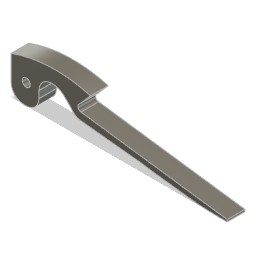
Fork v1 v14 (Autodesk Fusion 360 design; units mm, degrees)
Autodesk Fusion 360 part; units mm, degrees
derive "DerivedContext1" from "Forkzin v1"
sketch "Esboço1" plane through (0, 0, 0) normal (0, 1, 0) x (1, 0, 0)
  line L0 (0, 0) -> (100, 0)
  line L1 (100, 0) -> (100, 10)
  line L2 (100, 10) -> (0, 10)
  line L3 (0, 10) -> (0, 0)
  dimension "d1" = 100
  dimension "d2" = 10
  constraint horizontal L0
  constraint vertical L1
  constraint horizontal L2
  constraint vertical L3
  constraint coincident L0.start L3.end
  measures "d1" distance of L0.start L0.end
  measures "d2" distance of L0.start L2.end
extrude "Extrusão1" add sketch "Esboço1" along normal blind 15
sketch "Esboço2" plane through (0, 0, 0) normal (0, 0, 1) x (1, 0, 0)
  line L0 (0, 0) -> (100, 0)
  line L1 (100, 0) -> (100, 15)
  line L2 (100, 15) -> (0, 15)
  line L3 (0, 15) -> (0, 0)
  line L4 (0, 15) -> (25, 15)
  line L5 (25, 15) -> (35, 15)
  arc A0 (35, 15) -> (26.7898, 10.9801) centre (37.5, -0.5) ccw
  line L6 (27.6317, 8.7193) -> (100, 1)
  arc A1 (26.9383, 11.1168) -> (27.6317, 8.7193) centre (27.7747, 10.0597) ccw
  dimension "d5" = 10
  constraint coincident L2.end L3.start
  constraint coincident L2 L4.end
  constraint perpendicular L3 L4
  constraint perpendicular L3 L5
  constraint coincident L1 L6.end
  constraint tangent L6 A1
  constraint coincident A0 A1.start
  constraint coincident A1 A0.end
  measures "d5" distance of L4.end L5.end
extrude "Extrusão2" cut sketch "Esboço2" against normal blind 17 contours L1 L2 A0 L6 A1
sketch "Esboço3" plane through (0, 0, 0) normal (0, 0, 1) x (1, 0, 0)
  arc A0 (35, 15) -> (26.7898, 10.9801) centre (37.5, -0.5) ccw
  line L0 (35, 15) -> (0, 15)
  line L1 (0, 15) -> (0, 0)
  line L2 (0, 0) -> (100, 0)
  line L3 (100, 0) -> (100, 1)
  line L4 (100, 1) -> (27.6317, 8.7193)
  arc A1 (26.7898, 10.9801) -> (27.6317, 8.7193) centre (27.7747, 10.0597) ccw
  arc A2 (35, 15) -> (0, 15) centre (17.5, -32.5) ccw
  constraint coincident L0.end L1.start
  constraint coincident A0.start L0.start
extrude "Extrusão3" add sketch "Esboço3" against normal blind 10 contours L0 A2
extrude "Extrusão4" cut 1 faces at (13.4929, 9.1641, -10) along direction (0, 0, 1) blind 3
sketch "Esboço4" plane through (0, 0, 0) normal (0, 0, 1) x (1, 0, 0)
  arc A0 (35, 15) -> (26.7898, 10.9801) centre (37.5, -0.5) ccw
  arc A1 (35, 15) -> (0, 15) centre (17.5, -32.5) ccw
  line L0 (0, 15) -> (0, 0)
  line L1 (0, 0) -> (100, 0)
  line L2 (100, 0) -> (100, 1)
  line L3 (100, 1) -> (27.6317, 8.7193)
  arc A2 (26.7898, 10.9801) -> (27.6317, 8.7193) centre (27.7747, 10.0597) ccw
  arc A3 (27.2908, 11.4475) -> (26.7898, 10.9801) centre (30.4465, 7.5628) ccw
  line L4 (27.2908, 11.4475) -> (31.4325, 16.1661)
  constraint coincident A0.end A2.start
  constraint tangent A2 A3
  constraint coincident A1 L4.end
extrude "Extrusão5" cut sketch "Esboço4" against normal blind 12 contours A0 A1 A3 L4
sketch "Esboço5" plane through (0, 0, 0) normal (0, 0, 1) x (1, 0, 0)
  arc A0 (27.2908, 11.4475) -> (26.7898, 10.9801) centre (30.4465, 7.5628) ccw
  line L0 (27.2908, 11.4475) -> (31.4325, 16.1661)
  arc A1 (31.4325, 16.1661) -> (0, 15) centre (17.5, -32.5) ccw
  line L1 (0, 15) -> (0, 0)
  line L2 (0, 0) -> (100, 0)
  line L3 (100, 0) -> (100, 1)
  line L4 (100, 1) -> (27.6317, 8.7193)
  arc A2 (26.7898, 10.9801) -> (27.6317, 8.7193) centre (27.7747, 10.0597) ccw
  circle A3 centre (6, 8) radius 1.6
  line L5 (2.5, 2.5) -> (62.367, 2.5)
  line L6 (62.367, 2.5) -> (27.3666, 6.2334)
  arc A4 (24.9633, 12.6871) -> (27.3666, 6.2334) centre (27.7747, 10.0597) ccw
  arc A5 (25.5369, 13.239) -> (24.9633, 12.6871) centre (30.4465, 7.5628) ccw
  line L7 (25.5369, 13.239) -> (26.8268, 14.7086)
  arc A6 (26.8268, 14.7086) -> (2.5, 13.2236) centre (17.5, -32.5) ccw
  line L8 (2.5, 13.2236) -> (2.5, 2.5)
  dimension "d16" = -2.5
sketch "sketch 1220" plane through (-80, 0, 0) normal (0, 0, 1) x (1, 0, 0)
  line L0 (80, 0) -> (86, 0)
  line L1 (86, 0) -> (86, 8)
  circle A0 centre (86, 8) radius 1.6
extrude "Extrusão6" cut sketch "sketch 1220" against normal blind 14
sketch "Esboço6" plane through (0, 0, 0) normal (0, 0, 1) x (1, 0, 0)
  circle A0 centre (6, 8) radius 1.6
  arc A1 (27.2908, 11.4475) -> (26.7898, 10.9801) centre (30.4465, 7.5628) ccw
  line L0 (27.2908, 11.4475) -> (31.4325, 16.1661)
  arc A2 (31.4325, 16.1661) -> (0, 15) centre (17.5, -32.5) ccw
  line L1 (0, 15) -> (0, 0)
  line L2 (0, 0) -> (100, 0)
  line L3 (100, 0) -> (100, 1)
  line L4 (100, 1) -> (27.6317, 8.7193)
  arc A3 (26.7898, 10.9801) -> (27.6317, 8.7193) centre (27.7747, 10.0597) ccw
  line L5 (3, 3) -> (52.9655, 3)
  line L6 (52.9655, 3) -> (27.3135, 5.7362)
  arc A4 (24.598, 13.0285) -> (27.3135, 5.7362) centre (27.7747, 10.0597) ccw
  arc A5 (25.1834, 13.5942) -> (24.598, 13.0285) centre (30.4465, 7.5628) ccw
  line L7 (25.1834, 13.5942) -> (25.8725, 14.3794)
  arc A6 (25.8725, 14.3794) -> (15.2913, 15.0699) centre (17.5, -32.5) ccw
  line L8 (3, 12.8599) -> (3, 3)
  line L9 (6, 8) -> (11, 8)
  line L10 (11, 3) -> (11, 10.5747)
  arc A7 (15.2913, 15.0699) -> (11, 10.5747) centre (15.5, 10.5747) ccw
  dimension "d20" = 5
  dimension "d21" = 4.5
  constraint coincident A0.centre L9.start
  constraint parallel L2 L9
  constraint coincident L5 L10.start
  constraint perpendicular L9 L10
  constraint concentric A3 A4
  constraint concentric A1 A5
  constraint concentric A2 A6
  constraint tangent L6 A4
  constraint tangent A4 A5
  constraint tangent A6 A7
  constraint tangent L10 A7
  measures "d20" distance of A0.centre L9.end
  measures "d21" radius of A7
extrude "Extrusão8" cut sketch "Esboço6" against normal blind 9 contours L5 L6 A4 A5 L7 A6 L10 A7
sketch "Esboço7" plane through (0, 0, 0) normal (0, 0, 1) x (1, 0, 0)
  arc A0 (25.8725, 14.3794) -> (15.2913, 15.0699) centre (17.5, -32.5) ccw
  line L0 (25.8725, 14.3794) -> (25.1834, 13.5942)
  arc A1 (25.1834, 13.5942) -> (24.598, 13.0285) centre (30.4465, 7.5628) ccw
  arc A2 (24.598, 13.0285) -> (27.3135, 5.7362) centre (27.7747, 10.0597) ccw
  line L1 (27.3135, 5.7362) -> (52.9655, 3)
  line L2 (52.9655, 3) -> (11, 3)
  line L3 (11, 3) -> (11, 10.5747)
  arc A3 (15.2913, 15.0699) -> (11, 10.5747) centre (15.5, 10.5747) ccw
  circle A4 centre (6, 8) radius 1.6
  arc A5 (27.2908, 11.4475) -> (26.7898, 10.9801) centre (30.4465, 7.5628) ccw
  line L4 (27.2908, 11.4475) -> (31.4325, 16.1661)
  arc A6 (31.4325, 16.1661) -> (0, 15) centre (17.5, -32.5) ccw
  line L5 (0, 15) -> (0, 0)
  line L6 (0, 0) -> (100, 0)
  line L7 (100, 0) -> (100, 1)
  line L8 (100, 1) -> (27.6317, 8.7193)
  arc A7 (26.7898, 10.9801) -> (27.6317, 8.7193) centre (27.7747, 10.0597) ccw
extrude "Extrusão9" cut 1 faces at (24.9885, 3, -2.3333) along direction (0, -1, 0) blind 1
sketch "Esboço8" plane through (0, 0, 0) normal (0, 0, 1) x (1, 0, 0)
  arc A0 (27.2908, 11.4475) -> (26.7898, 10.9801) centre (30.4465, 7.5628) ccw
  line L0 (27.2908, 11.4475) -> (31.4325, 16.1661)
  arc A1 (31.4325, 16.1661) -> (0, 15) centre (17.5, -32.5) ccw
  line L1 (0, 15) -> (0, 0)
  line L2 (0, 0) -> (100, 0)
  line L3 (100, 0) -> (100, 1)
  line L4 (100, 1) -> (27.6317, 8.7193)
  arc A2 (26.7898, 10.9801) -> (27.6317, 8.7193) centre (27.7747, 10.0597) ccw
  circle A3 centre (6, 8) radius 1.6
  line L5 (52.9655, 3) -> (52.9655, 2)
  line L6 (52.9655, 2) -> (11, 2)
  line L7 (11, 2) -> (11, 10.5747)
  arc A4 (15.2913, 15.0699) -> (11, 10.5747) centre (15.5, 10.5747) ccw
  arc A5 (25.8725, 14.3794) -> (15.2913, 15.0699) centre (17.5, -32.5) ccw
  line L8 (25.8725, 14.3794) -> (25.1834, 13.5942)
  arc A6 (25.1834, 13.5942) -> (24.598, 13.0285) centre (30.4465, 7.5628) ccw
  arc A7 (24.598, 13.0285) -> (27.3135, 5.7362) centre (27.7747, 10.0597) ccw
  line L9 (27.3135, 5.7362) -> (52.9655, 3)
  arc A8 (27.359, 9.158) -> (26.9582, 8.7841) centre (29.8835, 6.0502) ccw
  line L10 (27.359, 9.158) -> (30.6723, 12.9328)
  arc A9 (30.6723, 12.9328) -> (5.5263, 12) centre (19.5263, -26) ccw
  line L11 (5.5263, 12) -> (5.5263, 0)
  line L12 (5.5263, 0) -> (85.5263, 0)
  line L13 (85.5263, 0) -> (85.5263, 0.8)
  line L14 (85.5263, 0.8) -> (27.6317, 6.9754)
  arc A10 (26.9582, 8.7841) -> (27.6317, 6.9754) centre (27.7461, 8.0477) ccw
  circle A11 centre (10.3263, 6.4) radius 1.28
  line L15 (47.8987, 2.4) -> (47.8987, 1.6)
  line L16 (47.8987, 1.6) -> (14.3263, 1.6)
  line L17 (14.3263, 1.6) -> (14.3263, 8.4598)
  arc A12 (17.7594, 12.0559) -> (14.3263, 8.4598) centre (17.9263, 8.4598) ccw
  arc A13 (26.2244, 11.5035) -> (17.7594, 12.0559) centre (19.5263, -26) ccw
  line L18 (26.2244, 11.5035) -> (25.6731, 10.8754)
  arc A14 (25.6731, 10.8754) -> (25.2047, 10.4228) centre (29.8835, 6.0502) ccw
  arc A15 (25.2047, 10.4228) -> (27.3772, 4.589) centre (27.7461, 8.0477) ccw
  line L19 (27.3772, 4.589) -> (47.8987, 2.4)
  line L20 (85.5263, 0.8) -> (27.6317, 8.7193)
  constraint coincident L13.end L14.start
  constraint coincident L4.end A2.end
extrude "Extrusão10" cut sketch "Esboço8" against normal blind 9 contours L2 L3 L4 L13 L20
sketch "Esboço9" plane through (0, 0, 0) normal (0, 0, 1) x (1, 0, 0)
  line L0 (85.5263, 0.8) -> (27.6317, 8.7193)
  arc A0 (26.7898, 10.9801) -> (27.6317, 8.7193) centre (27.7747, 10.0597) ccw
  arc A1 (27.2908, 11.4475) -> (26.7898, 10.9801) centre (30.4465, 7.5628) ccw
  line L1 (27.2908, 11.4475) -> (31.4325, 16.1661)
  arc A2 (31.4325, 16.1661) -> (0, 15) centre (17.5, -32.5) ccw
  line L2 (0, 15) -> (0, 0)
  line L3 (0, 0) -> (85.5263, 0)
  line L4 (85.5263, 0) -> (85.5263, 0.8)
  circle A3 centre (6, 8) radius 1.6
  line L5 (52.9655, 3) -> (52.9655, 2)
  line L6 (52.9655, 2) -> (11, 2)
  line L7 (11, 2) -> (11, 10.5747)
  arc A4 (15.2913, 15.0699) -> (11, 10.5747) centre (15.5, 10.5747) ccw
  arc A5 (25.8725, 14.3794) -> (15.2913, 15.0699) centre (17.5, -32.5) ccw
  line L8 (25.8725, 14.3794) -> (25.1834, 13.5942)
  arc A6 (25.1834, 13.5942) -> (24.598, 13.0285) centre (30.4465, 7.5628) ccw
  arc A7 (24.598, 13.0285) -> (27.3135, 5.7362) centre (27.7747, 10.0597) ccw
  line L9 (27.3135, 5.7362) -> (52.9655, 3)
  line L10 (50.639, 3.2482) -> (51.6246, 3.143)
  line L11 (52.9655, 2) -> (52.9655, 1.6515)
  line L12 (51.9946, 2) -> (50.5, 2)
  arc A8 (52.2592, 2.9243) -> (51.6246, 3.143) centre (51.4655, 1.6515) ccw
  arc A9 (51.9946, 2) -> (52.2592, 2.9243) centre (51.9946, 2.5) ccw
  dimension "d29" = 1.5
  dimension "d30" = 0.5
  constraint coincident L9 L10.start
  constraint parallel L9 L10
  constraint coincident L5.end L6.start
  constraint coincident L6 L12.end
  constraint perpendicular L5 L12
  constraint tangent L10 A8
  constraint tangent L11 A8
  constraint tangent L12 A9
  constraint tangent A8 A9
  measures "d29" radius of A8
  measures "d30" radius of A9
extrude "Extrusão11" add sketch "Esboço9" against normal blind 7 contours L5 L6 L9 A8 A9
fillet "Arredondamento1" radius 0.75 1 edges at (25.8725, 14.3794, -3.5)
fillet "Arredondamento2" radius 2 1 edges at (25.1834, 13.5942, -3.5)
sketch "Esboço10" plane through (0, 0, 0) normal (0, 0, 1) x (1, 0, 0)
  line L0 (85.5263, 0.8) -> (27.6317, 8.7193)
  arc A0 (26.7898, 10.9801) -> (27.6317, 8.7193) centre (27.7747, 10.0597) ccw
  arc A1 (27.2908, 11.4475) -> (26.7898, 10.9801) centre (30.4465, 7.5628) ccw
  line L1 (27.2908, 11.4475) -> (31.4325, 16.1661)
  arc A2 (31.4325, 16.1661) -> (0, 15) centre (17.5, -32.5) ccw
  line L2 (0, 15) -> (0, 0)
  line L3 (0, 0) -> (85.5263, 0)
  line L4 (85.5263, 0) -> (85.5263, 0.8)
  circle A3 centre (6, 8) radius 1.6
  arc A4 (52.2592, 2.9243) -> (51.6246, 3.143) centre (51.4655, 1.6515) ccw
  arc A5 (51.9946, 2) -> (52.2592, 2.9243) centre (51.9946, 2.5) ccw
  line L5 (51.9946, 2) -> (11, 2)
  line L6 (11, 2) -> (11, 10.5747)
  arc A6 (15.2913, 15.0699) -> (11, 10.5747) centre (15.5, 10.5747) ccw
  arc A7 (22.2936, 14.8793) -> (15.2913, 15.0699) centre (17.5, -32.5) ccw
  arc A8 (23.8826, 11.9979) -> (22.2936, 14.8793) centre (22.0923, 12.8894) ccw
  arc A9 (23.8826, 11.9979) -> (27.3135, 5.7362) centre (27.7747, 10.0597) ccw
  line L7 (27.3135, 5.7362) -> (51.6246, 3.143)
  line L8 (11, 2) -> (11, 0)
  line L9 (23.4407, 9.7105) -> (15.2913, 15.0699)
  line L10 (52.2592, 2.9243) -> (76, 0)
  line L11 (18.796, 12.7651) -> (11.5691, 12.7651)
  constraint coincident L5.end L6.start
  constraint coincident L3 L8.end
  constraint perpendicular L3 L8
  constraint coincident A9 L9.start
  constraint coincident A6.start A7.end
  constraint coincident A4.start A5.end
  constraint coincident L3 L10.end
  constraint coincident L9 L11.start
  constraint coincident A6 L11.end
  constraint horizontal L11
extrude "Extrusão12" cut sketch "Esboço10" against normal blind 14 contours L3 A5 L5 L8 L10
extrude "Extrusão13" add sketch "Esboço10" against normal blind 7 contours A7 A8 A9 L9
fillet "Arredondamento3" radius 3 1 edges at (15.2913, 15.0699, -3.5)
fillet "Arredondamento4" radius 35 1 edges at (23.4407, 9.7105, -3.5)
fillet "Arredondamento5" radius 102 1 edges at (76, 0, -3.5)
extrude "Extrusão14" cut sketch "Esboço10" against normal blind 15 contours A6 L9 L11
extrude "Extrusão15" add sketch "Esboço10" against normal blind 7 contours A6 L9 L11
fillet "Arredondamento6" radius 6.5 1 edges at (18.6632, 12.7651, -3.5)
fillet "Arredondamento7" radius 5 1 edges at (11.5691, 12.7651, -3.5)
fillet "Arredondamento8" radius 201 1 edges at (52.2592, 2.9243, -3.5)
fillet "Arredondamento9" radius 5 1 edges at (11, 0, -3.5)
fillet "Arredondamento10" radius 5 1 edges at (0, 0, -3.5)
